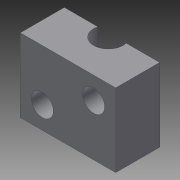
# Autodesk Inventor part: eye_cam_clamp
Saved by Autodesk Inventor 2015 (Build 190159000, 159)
## iProperties
Created: 2015-06-21
Part Number: eye_cam_clamp
Material: Generic
Document SubType Name: Modeling
Designer: Master
Density: 1 g/cm^3
Appearance: Default
Author: Master
Autodesk Inventor part; units mm, degrees
ref_plane "YZ Plane" through (0, 0, 0) normal (1, 0, 0) x (0, 1, 0)
ref_plane "XZ Plane" through (0, 0, 0) normal (0, 1, 0) x (-1, 0, 0)
ref_plane "XY Plane" through (0, 0, 0) normal (0, 0, 1) x (1, 0, 0)
sketch "Sketch1" plane through (0, 0, 0) normal (0, 0, 1) x (1, 0, 0)
  line L0 (-1.7679, 0.1299) -> (-1.7679, -25.6595) projected
  line L1 (-1.7679, -25.6595) -> (3, -25.6595) projected
  line L2 (3, -25.6595) -> (3, -15.6595) projected
  line L3 (3, -15.6595) -> (0, -15.6595) projected
  line L4 (0, -15.6595) -> (0, 0.1299) projected
  line L5 (-1.7679, 0.1299) -> (0, 0.1299) projected
  circle A0 centre (0, -18.6595) radius 1.5 projected
  line L6 (-5.2321, -25.6595) -> (-5.2321, 0.1299) projected
  line L7 (-10, 0.1299) -> (-5.2321, 0.1299) projected
  line L8 (-10, -25.6595) -> (-10, 0.1299) projected
  line L9 (-10, -25.6595) -> (-5.2321, -25.6595) projected
  circle A1 centre (-7, -22.6595) radius 1.5 projected
  line L10 (3, -25.6595) -> (-10, -25.6595)
  line L11 (-10, -25.6595) -> (-10, -15.6595)
  line L12 (-10, -15.6595) -> (3, -15.6595)
  line L13 (3, -15.6595) -> (3, -25.6595)
  point P0 (0, 0)
  constraints: 8 end point, 2 point on line
extrude "Extrusion1" add sketch "Sketch1" along normal blind 6 contours L12 L3 L2 L1 L0 | L0 L10 L6 L12 | L6 L9 L8 L12
sketch "Sketch2" plane through (-10, -25.6595, 0) normal (0, -1, 0) x (1, 0, 0)
  line L0 (0, 0) -> (13, 0) projected
  line L1 (13, 0) -> (13, 6) projected
  line L2 (0, 6) -> (13, 6) projected
  line L3 (0, 0) -> (0, 6) projected
  arc A0 (4.7679, 0) -> (8.2321, 0) centre (6.5, 1) ccw projected
  line L4 (0, 0) -> (4.7679, 0) projected
  line L5 (0, 0) -> (0, -4) projected
  line L6 (0, -4) -> (13, -4) projected
  line L7 (13, 0) -> (13, -4) projected
  line L8 (8.2321, 0) -> (13, 0) projected
  circle A1 centre (6.5, 0.5) radius 2
  point P0 (10, 0)
  dimension "d2" = 4
  dimension "d3" = 6.5
  dimension "d4" = 0.5
  constraints: 1 centre point
  measures "d2" diameter of A1
  measures "d3" distance from line of A1.centre L3
  measures "d4" distance of A0.centre A1.centre
extrude "Extrusion2" cut sketch "Sketch2" against normal through all contours L0 A1 | A0 L0 A1
body "Solid1"
